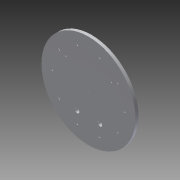
# Autodesk Inventor part: Grundplatte
Saved by Autodesk Inventor 2015 (Build 190159000, 159)
## iProperties
Created: 2018-03-07
Part Number: Grundplatte
Material: Generisch
Document SubType Name: Modeling
Designer: wepet
Density: 1 g/cm^3
Appearance: Vorgabe
Author: wepet
Autodesk Inventor part; units mm, degrees
ref_plane "YZ Plane" through (0, 0, 0) normal (1, 0, 0) x (0, 1, 0)
ref_plane "XZ Plane" through (0, 0, 0) normal (0, 1, 0) x (-1, 0, 0)
ref_plane "XY Plane" through (0, 0, 0) normal (0, 0, 1) x (1, 0, 0)
sketch "Skizze1" plane through (0, 0, 0) normal (0, 1, 0) x (-1, 0, 0)
  circle A0 centre (0, 0) radius 247.5
  dimension "d0" = 495
  constraints: 1 centre point, 1 coincident
  measures "d0" diameter of A0
extrude "Extrusion_grundplatte" add sketch "Skizze1" along normal blind 16
sketch "Skizze2" plane through (0, 16, 0) normal (0, 1, 0) x (1, 0, 0)
  circle A0 centre (0, 0) radius 247.5 projected
  line L0 (-45, 220) -> (45, 220) construction
  line L1 (45, 220) -> (45, 190) construction
  line L2 (45, 190) -> (-45, 190) construction
  line L3 (-45, 190) -> (-45, 220) construction
  line L4 (0, 190) -> (0, 220) construction
  line L5 (-32.5, 205) -> (32.5, 205) construction
  line L6 (0, 0) -> (0, 220) construction
  line L7 (-165.7185, 151.5334) -> (-92.907, 204.4341) construction
  line L8 (-92.907, 204.4341) -> (-75.2734, 180.1636) construction
  line L9 (-75.2734, 180.1636) -> (-148.085, 127.2629) construction
  line L10 (-148.085, 127.2629) -> (-165.7185, 151.5334) construction
  line L11 (-111.6792, 153.7132) -> (-129.3128, 177.9837) construction
  line L12 (-146.789, 146.7455) -> (-94.2029, 184.9515) construction
  line L13 (-223.1382, 25.1862) -> (-195.3267, 110.7813) construction
  line L14 (-195.3267, 110.7813) -> (-166.795, 101.5108) construction
  line L15 (-166.795, 101.5108) -> (-194.6065, 15.9157) construction
  line L16 (-194.6065, 15.9157) -> (-223.1382, 25.1862) construction
  line L17 (-180.7007, 58.7132) -> (-209.2324, 67.9837) construction
  line L18 (-205.0096, 32.4391) -> (-184.9235, 94.2578) construction
  line L19 (-195.3267, -110.7813) -> (-223.1382, -25.1862) construction
  line L20 (-223.1382, -25.1862) -> (-194.6065, -15.9157) construction
  line L21 (-194.6065, -15.9157) -> (-166.795, -101.5108) construction
  line L22 (-166.795, -101.5108) -> (-195.3267, -110.7813) construction
  line L23 (-180.7007, -58.7132) -> (-209.2324, -67.9837) construction
  line L24 (-184.9235, -94.2578) -> (-205.0096, -32.4391) construction
  line L25 (-92.907, -204.4341) -> (-165.7185, -151.5334) construction
  line L26 (-165.7185, -151.5334) -> (-148.085, -127.2629) construction
  line L27 (-148.085, -127.2629) -> (-75.2734, -180.1636) construction
  line L28 (-75.2734, -180.1636) -> (-92.907, -204.4341) construction
  line L29 (-111.6792, -153.7132) -> (-129.3128, -177.9837) construction
  line L30 (-94.2029, -184.9515) -> (-146.789, -146.7455) construction
  line L31 (45, -220) -> (-45, -220) construction
  line L32 (-45, -220) -> (-45, -190) construction
  line L33 (-45, -190) -> (45, -190) construction
  line L34 (45, -190) -> (45, -220) construction
  line L35 (0, -190) -> (0, -220) construction
  line L36 (32.5, -205) -> (-32.5, -205) construction
  line L37 (165.7185, -151.5334) -> (92.907, -204.4341) construction
  line L38 (92.907, -204.4341) -> (75.2734, -180.1636) construction
  line L39 (75.2734, -180.1636) -> (148.085, -127.2629) construction
  line L40 (148.085, -127.2629) -> (165.7185, -151.5334) construction
  line L41 (111.6792, -153.7132) -> (129.3128, -177.9837) construction
  line L42 (146.789, -146.7455) -> (94.2029, -184.9515) construction
  line L43 (223.1382, -25.1862) -> (195.3267, -110.7813) construction
  line L44 (195.3267, -110.7813) -> (166.795, -101.5108) construction
  line L45 (166.795, -101.5108) -> (194.6065, -15.9157) construction
  line L46 (194.6065, -15.9157) -> (223.1382, -25.1862) construction
  line L47 (180.7007, -58.7132) -> (209.2324, -67.9837) construction
  line L48 (205.0096, -32.4391) -> (184.9235, -94.2578) construction
  line L49 (195.3267, 110.7813) -> (223.1382, 25.1862) construction
  line L50 (223.1382, 25.1862) -> (194.6065, 15.9157) construction
  line L51 (194.6065, 15.9157) -> (166.795, 101.5108) construction
  line L52 (166.795, 101.5108) -> (195.3267, 110.7813) construction
  line L53 (180.7007, 58.7132) -> (209.2324, 67.9837) construction
  line L54 (184.9235, 94.2578) -> (205.0096, 32.4391) construction
  line L55 (92.907, 204.4341) -> (165.7185, 151.5334) construction
  line L56 (165.7185, 151.5334) -> (148.085, 127.2629) construction
  line L57 (148.085, 127.2629) -> (75.2734, 180.1636) construction
  line L58 (75.2734, 180.1636) -> (92.907, 204.4341) construction
  line L59 (111.6792, 153.7132) -> (129.3128, 177.9837) construction
  line L60 (94.2029, 184.9515) -> (146.789, 146.7455) construction
  point P0 (35, 190)
  point P1 (-35, 190)
  point P2 (0, 205)
  point P3 (-83.3636, 174.2857)
  point P4 (-139.9948, 133.1407)
  point P5 (-120.496, 165.8485)
  point P6 (-169.8851, 92.0002)
  point P7 (-191.5163, 25.4263)
  point P8 (-194.9666, 63.3485)
  point P9 (-191.5163, -25.4263)
  point P10 (-169.8851, -92.0002)
  point P11 (-194.9666, -63.3485)
  point P12 (-139.9948, -133.1407)
  point P13 (-83.3636, -174.2857)
  point P14 (-120.496, -165.8485)
  point P15 (-35, -190)
  point P16 (35, -190)
  point P17 (0, -205)
  point P18 (83.3636, -174.2857)
  point P19 (139.9948, -133.1407)
  point P20 (120.496, -165.8485)
  point P21 (169.8851, -92.0002)
  point P22 (191.5163, -25.4263)
  point P23 (194.9666, -63.3485)
  point P24 (191.5163, 25.4263)
  point P25 (169.8851, 92.0002)
  point P26 (194.9666, 63.3485)
  point P27 (139.9948, 133.1407)
  point P28 (83.3636, 174.2857)
  point P29 (120.496, 165.8485)
  dimension "d3" = 90
  dimension "d4" = 30
  dimension "d5" = 35
  dimension "d6" = 35
  dimension "d7" = 32.5
  dimension "d8" = 32.5
  dimension "d9" = 220
  dimension "d12" = 360
  constraints: 122 end point, 20 point on line, 13 midpoint, 3 perpendicular, 2 horizontal, 1 vertical, 171 other
  measures "d3" distance of L0.end L0.start
  measures "d4" distance of L2.end L0.start
  measures "d5" distance of point (-35, 190) L4.start
  measures "d6" distance from line of L4 point (35, 190)
  measures "d7" distance from line of L4 L5.end
  measures "d8" distance from line of L4 L5.start
  measures "d9" distance of L6.start L4.end
hole "Bohrung_leds" at (35, 16, -190) at (-35, 16, -190) at (-45, 16, -220) at (45, 16, -220) at (-165.7185, 16, -151.5334) at (-92.907, 16, -204.4341) at (-139.9948, 16, -133.1407) at (-83.3636, 16, -174.2857) at (-223.1382, 16, -25.1862) at (-195.3267, 16, -110.7813) at (-191.5163, 16, -25.4263) at (-169.8851, 16, -92.0002) at (-195.3267, 16, 110.7813) at (-223.1382, 16, 25.1862) at (-169.8851, 16, 92.0002) at (-191.5163, 16, 25.4263) at (-92.907, 16, 204.4341) at (-165.7185, 16, 151.5334) at (-83.3636, 16, 174.2857) at (-139.9948, 16, 133.1407) at (45, 16, 220) at (-45, 16, 220) at (35, 16, 190) at (-35, 16, 190) at (165.7185, 16, 151.5334) at (92.907, 16, 204.4341) at (139.9948, 16, 133.1407) at (83.3636, 16, 174.2857) at (223.1382, 16, 25.1862) at (195.3267, 16, 110.7813) at (191.5163, 16, 25.4263) at (169.8851, 16, 92.0002) at (195.3267, 16, -110.7813) at (223.1382, 16, -25.1862) at (169.8851, 16, -92.0002) at (191.5163, 16, -25.4263) at (92.907, 16, -204.4341) at (165.7185, 16, -151.5334) at (83.3636, 16, -174.2857) at (139.9948, 16, -133.1407) direction (0, -1, 0) diameter 2 depth 10 tip angle 118
sketch "Skizze3" plane through (0, 16, 0) normal (0, 1, 0) x (1, 0, 0)
  circle A0 centre (83.3636, 174.2857) radius 1 projected
  circle A1 centre (92.907, 204.4341) radius 1 projected
  circle A2 centre (169.8851, 92.0002) radius 1 projected
  circle A3 centre (195.3267, 110.7813) radius 1 projected
  circle A4 centre (191.5163, -25.4263) radius 1 projected
  circle A5 centre (223.1382, -25.1862) radius 1 projected
  circle A6 centre (139.9948, -133.1407) radius 1 projected
  circle A7 centre (165.7185, -151.5334) radius 1 projected
  circle A8 centre (35, -190) radius 1 projected
  circle A9 centre (45, -220) radius 1 projected
  circle A10 centre (-83.3636, -174.2857) radius 1 projected
  circle A11 centre (-92.907, -204.4341) radius 1 projected
  circle A12 centre (-169.8851, -92.0002) radius 1 projected
  circle A13 centre (-195.3267, -110.7813) radius 1 projected
  circle A14 centre (-191.5163, 25.4263) radius 1 projected
  circle A15 centre (-223.1382, 25.1862) radius 1 projected
  circle A16 centre (-139.9948, 133.1407) radius 1 projected
  circle A17 centre (-165.7185, 151.5334) radius 1 projected
  circle A18 centre (-45, 220) radius 1 projected
  circle A19 centre (35, 190) radius 1 projected
  circle A20 centre (-35, 190) radius 1 projected
  circle A21 centre (45, 220) radius 1 projected
  circle A22 centre (-92.907, 204.4341) radius 1 projected
  circle A23 centre (-83.3636, 174.2857) radius 1 projected
  circle A24 centre (-195.3267, 110.7813) radius 1 projected
  circle A25 centre (-169.8851, 92.0002) radius 1 projected
  circle A26 centre (-223.1382, -25.1862) radius 1 projected
  circle A27 centre (-191.5163, -25.4263) radius 1 projected
  circle A28 centre (-165.7185, -151.5334) radius 1 projected
  circle A29 centre (-139.9948, -133.1407) radius 1 projected
  circle A30 centre (-45, -220) radius 1 projected
  circle A31 centre (-35, -190) radius 1 projected
  circle A32 centre (92.907, -204.4341) radius 1 projected
  circle A33 centre (83.3636, -174.2857) radius 1 projected
  circle A34 centre (195.3267, -110.7813) radius 1 projected
  circle A35 centre (169.8851, -92.0002) radius 1 projected
  circle A36 centre (223.1382, 25.1862) radius 1 projected
  circle A37 centre (191.5163, 25.4263) radius 1 projected
  circle A38 centre (165.7185, 151.5334) radius 1 projected
  circle A39 centre (139.9948, 133.1407) radius 1 projected
  circle A40 centre (0, 0) radius 247.5 projected
  circle A41 centre (0, 0) radius 247.5 projected
  line L0 (60, 120) -> (-60, 120) construction
  line L1 (0, 0) -> (0, 120) construction
  dimension "d71" = 100
  dimension "d21" = 120
  dimension "d22" = 120
  constraints: 4 end point, 2 midpoint, 1 horizontal, 1 perpendicular, 1 point on line
  measures "d21" distance of L1.start L1.end
  measures "d22" distance of L0.start L0.end
hole "Bohrung_extern" at (60, 16, -120) at (-60, 16, -120) direction (0, -1, 0) diameter 24 end through all
sketch "Skizze4" plane through (0, 16, 0) normal (0, 1, 0) x (1, 0, 0)
  circle A0 centre (0, 0) radius 247.5 projected
  line L0 (45, -35) -> (-45, -35) construction
  line L1 (-45, -35) -> (-45, 35) construction
  line L2 (-45, 35) -> (45, 35) construction
  line L3 (45, 35) -> (45, -35) construction
  line L4 (0, 0) -> (0, -35) construction
  dimension "d30" = 70
  dimension "d31" = 90
  dimension "d32" = 35
  constraints: 11 end point, 4 coincident, 2 parallel, 2 perpendicular, 1 horizontal, 1 midpoint
  measures "d30" distance of L0.end L1.end
  measures "d31" distance of L0.start L0.end
  measures "d32" distance of L4.start L4.end
hole "Bohrung_mcu" at (-45, 16, 35) at (-45, 16, -35) at (45, 16, -35) at (45, 16, 35) direction (0, -1, 0) diameter 2 depth 10 tip angle 118
sketch "Skizze5" plane through (0, 16, 0) normal (0, 1, 0) x (1, 0, 0)
  circle A0 centre (0, 0) radius 247.5 construction
  line L0 (120, -100) -> (-120, -100) construction
  circle A1 centre (60, 120) radius 12 projected
  circle A2 centre (-60, 120) radius 12 projected
  circle A3 centre (60, 120) radius 12 projected
  line L1 (0, 0) -> (0, -100) construction
  dimension "d71" = 100
  dimension "d72" = 240
  constraints: 6 end point, 2 coincident, 1 horizontal, 1 midpoint, 1 vertical
  measures "d71" distance of L1.start L1.end
  measures "d72" distance of L0.start L0.end
hole "Bohrung_taster" at (120, 16, 100) at (-120, 16, 100) direction (0, -1, 0) diameter 7 end through all counterbore diameter 10 counterbore depth 12
sketch "Skizze6" plane through (0, 0, 0) normal (0, -1, 0) x (1, 0, 0)
  line L0 (0, 0) -> (190, 0) construction
  circle A0 centre (0, 0) radius 247.5 projected
  point P0 (153.7132, 111.6792)
  point P1 (153.7132, 111.6792)
  point P2 (58.7132, 180.7007)
  point P3 (58.7132, 180.7007)
  point P4 (-58.7132, 180.7007)
  point P5 (-58.7132, 180.7007)
  point P6 (-153.7132, 111.6792)
  point P7 (-153.7132, 111.6792)
  point P8 (-190, 0)
  point P9 (-190, 0)
  point P10 (-153.7132, -111.6792)
  point P11 (-153.7132, -111.6792)
  point P12 (-58.7132, -180.7007)
  point P13 (-58.7132, -180.7007)
  point P14 (58.7132, -180.7007)
  point P15 (58.7132, -180.7007)
  point P16 (153.7132, -111.6792)
  point P17 (153.7132, -111.6792)
  dimension "d50" = 360
  dimension "d59" = 190
  dimension "d62" = 360
  constraints: 11 coincident, 2 end point, 1 horizontal, 21 other
  measures "d59" distance of L0.start L0.end
hole "Bohrung_halter_plexiglas" at (190, 0, 0) at (153.7132, 0, 111.6792) at (58.7132, 0, 180.7007) at (-58.7132, 0, 180.7007) at (-153.7132, 0, 111.6792) at (-190, 0, 0) at (-153.7132, 0, -111.6792) at (-58.7132, 0, -180.7007) at (58.7132, 0, -180.7007) at (153.7132, 0, -111.6792) direction (0, 1, 0) diameter 4 end through all counterbore diameter 9 counterbore depth 4
sketch "Skizze7" plane through (0, 0, 0) normal (0, -1, 0) x (1, 0, 0)
  circle A0 centre (0, 0) radius 247.5 projected
  constraints: 1 coincident
hole "Bohrung6" at (0, 0, 0) direction (0, 1, 0) diameter 3 end through all
